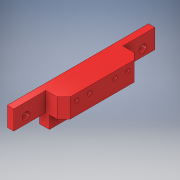
# Autodesk Inventor part: КВ33.044.202
Saved by Autodesk Inventor 2019 (Build 230136000, 136)
## iProperties
Created: 2019-07-15
Part Number: КВ33.044.202
Material: Пластик АБС
Document SubType Name: Modeling
Designer: Петров Иван
Density: 1.06 g/cm^3
Appearance: Светло-красный
Description: Фиксатор каретки
Author: Петров Иван
Autodesk Inventor part; units mm, degrees
ref_plane "YZ Plane" through (0, 0, 0) normal (1, 0, 0) x (0, 1, 0)
ref_plane "XZ Plane" through (0, 0, 0) normal (0, 1, 0) x (-1, 0, 0)
ref_plane "XY Plane" through (0, 0, 0) normal (0, 0, 1) x (1, 0, 0)
sketch "Эскиз1" plane through (0, 0, 0) normal (1, 0, 0) x (0, 1, 0)
  line L0 (-5, 0) -> (0, 0)
  line L1 (0, 0) -> (0, -10)
  line L2 (0, -10) -> (0, 0)
  line L3 (0, 0) -> (0, 10)
  circle A0 centre (0, -10) radius 1.75
  line L4 (0, -10) -> (0, -20)
  circle A1 centre (0, -20) radius 1.75
  circle A2 centre (0, 10) radius 1.75
  line L5 (0, 10) -> (0, 20)
  circle A3 centre (0, 20) radius 1.75
  line L6 (-10, 25) -> (5, 25)
  line L7 (5, 25) -> (5, -25)
  line L8 (5, -25) -> (-10, -25)
  line L9 (-10, -25) -> (-10, 25)
  line L10 (-10, 25) -> (5, -25) construction
  line L11 (5, 25) -> (-10, -25) construction
  point P0 (0, 0)
  point P1 (0, 0)
  dimension "d0" = 5
  dimension "d1" = 10
  dimension "d2" = 10
  dimension "d3" = 3.5
  dimension "d4" = 10
  dimension "d5" = 3.5
  dimension "d6" = 3.5
  dimension "d7" = 10
  dimension "d8" = 3.5
  dimension "d9" = 15
  dimension "d10" = 50
  constraints: 24 end point, 4 centre point, 4 coincident, 3 equal length, 2 perpendicular, 1 horizontal, 1 point on line
  measures "d0" distance of L0.start L0.end
  measures "d1" distance of L0.end L1.end
  measures "d2" distance of L0.end L3.end
  measures "d3" diameter of A0
  measures "d4" distance of L4.start L4.end
  measures "d5" diameter of A1
  measures "d6" diameter of A2
  measures "d7" distance of L5.start L5.end
  measures "d8" diameter of A3
  measures "d9" distance of L7.end L8.end
  measures "d10" distance of L6.end L7.end
extrude "Выдавливание1" add sketch "Эскиз1" along normal blind 6
sketch "Эскиз3" plane through (0, 0, 0) normal (-1, 0, 0) x (0, 0, 1)
  line L0 (-5, -5) -> (5, -5)
  line L1 (5, -5) -> (5, 5)
  line L2 (5, 5) -> (-5, 5)
  line L3 (-5, 5) -> (-5, -5)
  line L4 (-5, -5) -> (5, 5) construction
  line L5 (5, -5) -> (-5, 5) construction
  point P0 (0, 0)
  dimension "d17" = 10
  dimension "d18" = 10
  constraints: 12 end point, 2 midpoint, 2 parallel, 1 horizontal, 1 perpendicular
  measures "d17" distance of L2.end L1.end
  measures "d18" distance of L1.end L0.end
extrude "Выдавливание3" add sketch "Эскиз3" along normal blind 4.9
sketch "Эскиз5" plane through (0, -5, -5) normal (0, -1, 0) x (1, 0, 0)
  line L0 (-12.9, 0) -> (-12.9, 10) projected
  line L1 (-12.9, 0) -> (-5.1, 0)
  line L2 (-5.1, 0) -> (-5.1, 10)
  line L3 (-5.1, 10) -> (-12.9, 10)
  line L4 (-12.9, 10) -> (-12.9, 0)
  point P0 (0, 5)
  dimension "d26" = 7.8
  constraints: 8 end point, 2 parallel, 1 horizontal, 1 perpendicular
  measures "d26" distance of L3.end L2.end
extrude "Выдавливание4" add sketch "Эскиз5" along normal blind 15
move faces "Перенос1" translate (-8, 0, 0) faces at (-4.9, 1.6667, -1.6667)
move faces "Перенос3" translate (0, 0, 5) faces at (2, -5, 25)
sketch "Эскиз7" plane through (0, 0, 0) normal (-1, 0, 0) x (0, 0, 1)
  line L0 (30, 5) -> (30, -10) projected
  line L1 (30, 5) -> (25, 5)
  line L2 (25, 5) -> (25, -10)
  line L3 (25, -10) -> (30, -10)
  line L4 (30, -10) -> (30, 5)
  point P0 (0, 0)
  dimension "d42" = 5
  dimension "d43" = 15
  constraints: 8 end point, 2 parallel, 1 horizontal, 1 perpendicular
  measures "d42" distance of L3.end L2.end
  measures "d43" distance of L2.end L1.end
extrude "Выдавливание6" add sketch "Эскиз7" along normal up to surface (12.9 mm away)
chamfer "Фаска1" distance 5 angle 45 1 edges at (6, -2.5, 30)
sketch "Эскиз8" plane through (-12.9, -10, 30) normal (0, 0, 1) x (1, 0, 0)
  line L0 (0, 15) -> (0, 0) projected
  line L1 (0, 15) -> (5, 15)
  line L2 (5, 15) -> (5, 0)
  line L3 (5, 0) -> (0, 0)
  line L4 (0, 0) -> (0, 15)
  point P0 (12.9, 10)
  dimension "d49" = 5
  dimension "d50" = 15
  constraints: 8 end point, 2 parallel, 1 horizontal, 1 perpendicular
  measures "d49" distance of L2.end L3.end
  measures "d50" distance of L1.end L2.end
extrude "Выдавливание7" add sketch "Эскиз8" along normal blind 25
sketch "Эскиз9" plane through (-12.9, -10, 25) normal (-1, 0, 0) x (0, 0, 1)
  line L0 (30, 0) -> (30, 15) projected
  circle A0 centre (20.5, 5.5) radius 3
  line L1 (0, 15) -> (30, 15) projected
  point P0 (-25, 10)
  dimension "d54" = 6
  dimension "d57" = 9.5
  constraints: 1 centre point
  measures "d54" diameter of A0
  measures "d57" distance from line of L1 A0.centre
extrude "Выдавливание8" cut sketch "Эскиз9" against normal blind 25
move faces "Перенос4" translate (0, 0, -5) faces at (2, 0, -25)
sketch "Эскиз10" plane through (0, 0, 0) normal (-1, 0, 0) x (0, 0, 1)
  line L0 (-30, 5) -> (25, 5) projected
  line L1 (-30, 5) -> (-25, 5)
  line L2 (-25, 5) -> (-25, -10)
  line L3 (-25, -10) -> (-30, -10)
  line L4 (-30, -10) -> (-30, 5)
  point P0 (0, 0)
  dimension "d64" = 5
  dimension "d65" = 15
  constraints: 8 end point, 2 parallel, 1 horizontal, 1 perpendicular
  measures "d64" distance of L2.end L3.end
  measures "d65" distance of L1.end L2.end
extrude "Выдавливание9" add sketch "Эскиз10" along normal up to surface (12.9 mm away)
sketch "Эскиз11" plane through (6, -10, -30) normal (0, 0, -1) x (-1, 0, 0)
  line L0 (18.9, 15) -> (18.9, 0) projected
  line L1 (18.9, 15) -> (13.9, 15)
  line L2 (13.9, 15) -> (13.9, 0)
  line L3 (13.9, 0) -> (18.9, 0)
  line L4 (18.9, 0) -> (18.9, 15)
  point P0 (6, 10)
  dimension "d68" = 5
  dimension "d69" = 15
  constraints: 8 end point, 2 parallel, 1 horizontal, 1 perpendicular
  measures "d68" distance of L3.end L2.end
  measures "d69" distance of L2.end L1.end
extrude "Выдавливание10" add sketch "Эскиз11" along normal blind 25
sketch "Эскиз12" plane through (-12.9, -10, -25) normal (-1, 0, 0) x (0, 0, 1)
  circle A0 centre (-20.5, 5.5) radius 3
  line L0 (0, 15) -> (-30, 15) projected
  line L1 (-30, 0) -> (-30, 15) projected
  point P0 (25, 10)
  dimension "d72" = 6
  dimension "d73" = 9.5
  dimension "d74" = 9.5
  constraints: 1 centre point
  measures "d72" diameter of A0
  measures "d73" distance from line of L0 A0.centre
  measures "d74" distance from line of L1 A0.centre
extrude "Выдавливание11" cut sketch "Эскиз12" against normal blind 25
chamfer "Фаска4" distance 5 angle 45 1 edges at (6, -2.5, -30)
move faces "Перенос5" translate (-12.9, 0, 0) faces at (0, -8.3333, 1.6667)
sketch "Эскиз14" plane through (-12.9, -10, -55) normal (-1, 0, 0) x (0, 0, 1)
  circle A0 centre (75, 10) radius 1.75 projected
  circle A1 centre (75, 10) radius 3.5
  circle A2 centre (65, 10) radius 1.75 projected
  circle A3 centre (65, 10) radius 3.5
  circle A4 centre (45, 10) radius 1.75 projected
  circle A5 centre (45, 10) radius 3.5
  circle A6 centre (35, 10) radius 1.75 projected
  circle A7 centre (35, 10) radius 3.5
  point P0 (55, 10)
  dimension "d95" = 7
  dimension "d96" = 7
  dimension "d97" = 7
  dimension "d98" = 7
  constraints: 4 centre point, 4 coincident
  measures "d95" diameter of A1
  measures "d96" diameter of A3
  measures "d97" diameter of A5
  measures "d98" diameter of A7
extrude "Выдавливание13" cut sketch "Эскиз14" against normal blind 12.9
move faces "Перенос6" translate (0, 0, -25) faces at (-7.7, -13.3333, -5)
move faces "Перенос7" translate (0, 0, 25) faces at (-7.7, -16.6667, 5)
equation "\"d1\" = d2"
equation "\"d3\" = d5"
equation "\"d4\" = d2"
equation "\"d6\" = d5"
equation "\"d7\" = d2"
equation "\"d8\" = d5"
equation "\"d96\" = d95"
equation "\"d97\" = d95"
equation "\"d98\" = d95"
